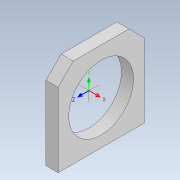
# Autodesk Inventor part: body_motor_fix_board_right
Saved by Autodesk Inventor 2020 (Build 240168000, 168)
## iProperties
Created: 2021-01-12
Part Number: body_motor_fix_board_right
Material: Generic
Document SubType Name: Modeling
Designer: DELL
Density: 1 g/cm^3
Appearance: Default
Author: DELL
Autodesk Inventor part; units mm, degrees
ref_plane "YZ Plane" through (0, 0, 0) normal (1, 0, 0) x (0, 1, 0)
ref_plane "XZ Plane" through (0, 0, 0) normal (0, 1, 0) x (-1, 0, 0)
ref_plane "XY Plane" through (0, 0, 0) normal (0, 0, 1) x (1, 0, 0)
sketch "Sketch1" plane through (0, 0, 0) normal (1, 0, 0) x (0, 1, 0)
  circle A0 centre (0, 0) radius 32
  line L0 (45, 42.5) -> (-43, 42.5)
  line L1 (-43, 42.5) -> (-43, -42.5)
  line L2 (-43, -42.5) -> (45, -42.5)
  line L3 (45, -42.5) -> (45, 42.5)
  line L4 (45, 42.5) -> (-43, -42.5) construction
  line L5 (-43, 42.5) -> (45, -42.5) construction
  line L6 (30, 42.5) -> (45, 27.5)
  line L7 (45, -27.5) -> (30, -42.5)
  line L8 (-43, 0) -> (45, 0) construction
  point P0 (1, 0)
  point P1 (1, 0)
  dimension "d0" = 64
  dimension "d1" = 88
  dimension "d2" = 43
  dimension "d3" = 85
  dimension "d4" = 15
  dimension "d5" = 45
  constraints: 18 end point, 5 midpoint, 4 point on line, 3 perpendicular, 2 parallel, 1 centre point, 1 coincident, 1 horizontal, 1 horizontal alignment
  measures "d0" diameter of A0
  measures "d1" distance between parallel lines of L3 L1
  measures "d2" distance from line of L1 A0.centre
  measures "d3" distance between parallel lines of L2 L0
  measures "d4" distance of L0.start L6.end
  measures "d5" angle of L3 L6
extrude "Extrusion1" add sketch "Sketch1" along normal blind 12 contours L6 L3 L7 L2 L1 L0
body "Solid1"
